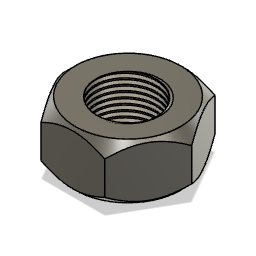
HEX NUT (Autodesk Fusion 360 design; units mm, degrees)
Autodesk Fusion 360 part; units mm, degrees
sketch "Sketch1" plane through (0, 0, 0) normal (0, 1, 0) x (1, 0, 0)
  line L0 (5.7735, -10) -> (11.547, 0)
  line L1 (11.547, 0) -> (5.7735, 10)
  line L2 (5.7735, 10) -> (-5.7735, 10)
  line L3 (-5.7735, 10) -> (-11.547, 0)
  line L4 (-11.547, 0) -> (-5.7735, -10)
  line L5 (-5.7735, -10) -> (5.7735, -10)
  dimension "d1" = 10
  measures "d1" distance of origin L5
extrude "Extrude1" add sketch "Sketch1" along normal blind 10
sketch "Sketch2" plane through (0, 0, 0) normal (0, 0, 1) x (1, 0, 0)
  line L0 (11.5475, 10) -> (9.5475, 10)
  line L1 (11.5475, 10) -> (11.5475, 8)
  line L2 (11.5475, 8) -> (9.5475, 10)
  dimension "d4" = 2
  dimension "d5" = 2
  constraint horizontal L0
  constraint perpendicular L0 L1
  measures "d4" distance of L0.start L0.end
  measures "d5" distance of L0.start L1.end
revolve "Revolve1" cut sketch "Sketch2" angle 360 about axis through (0, 1.75, 0) along (0, 1, 0)
ref_plane "WorkPlane1" through (0, 5, 0) normal (0, 1, 0) x (0, 0, 1)
mirror "Mirror1" about plane through (0, 5, 0) normal (0, 1, 0) of "Revolve1"
hole "Hole1" at (-0.0958, 0, 0.1437) direction (0, 1, 0) diameter 11.035 depth 10 tip angle 180 countersink diameter 12 countersink angle 90
thread "Thread1" "GB Metric profile 12.0 M12x1 6H" major diameter 12.152 minor diameter 11.035 pitch 1 angle 60 modelled right hand crest width 0.2719 on face at (0.1792, 3.655, -5.3669) crest through (-0.0958, 0.7325, -5.3738)
